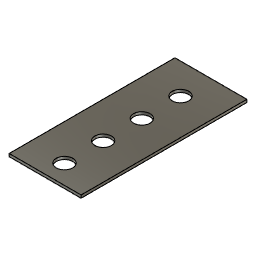
Untitled v1 (Autodesk Fusion 360 design; units mm, degrees)
Autodesk Fusion 360 part; units mm, degrees
sketch "Sketch1" plane through (0, 0, 0) normal (0, 0, 1) x (1, 0, 0)
  line L0 (6.508, 15) -> (-6.508, 15)
  line L1 (-6.508, 15) -> (-6.508, -15)
  line L2 (-6.508, -15) -> (6.508, -15)
  line L3 (6.508, -15) -> (6.508, 15)
  line L4 (6.508, 15) -> (-6.508, -15) construction
  line L5 (-6.508, 15) -> (6.508, -15) construction
  line L6 (0, 15) -> (0, -15) construction
  circle A0 centre (0, 13) radius 2
  circle A1 centre (0, 9.5) radius 1.5
  circle A2 centre (0, 6) radius 2
  circle A3 centre (0, 2.5) radius 1.5
  circle A4 centre (0, -1) radius 2
  circle A5 centre (0, -4.5) radius 1.5
  circle A6 centre (0, -8) radius 2
  circle A7 centre (0, -11.5) radius 1.5
  dimension "d1" = 13.016
  dimension "d2" = 30
  dimension "d3" = 4
  dimension "d4" = 3
  dimension "d5" = 4
  dimension "d6" = 3
  dimension "d7" = 4
  dimension "d8" = 3
  dimension "d9" = 4
  dimension "d10" = 3
  constraint horizontal L0
  constraint perpendicular L0 L1
  constraint parallel L0 L2
  constraint parallel L1 L3
  constraint coincident L4 origin
  constraint coincident L5 origin
  constraint midpoint L0 L6.start
  constraint midpoint L2 L6.end
  constraint coincident L6.start A0
  measures "d1" distance of L1.end L2.end
  measures "d2" distance of L0.end L1.end
  measures "d3" diameter of A0
  measures "d4" diameter of A1
  measures "d5" diameter of A2
  measures "d6" diameter of A3
  measures "d7" diameter of A4
  measures "d8" diameter of A5
  measures "d9" diameter of A6
  measures "d10" diameter of A7
extrude "Extrude1" add sketch "Sketch1" along normal blind 0.5 contours A6 | A4 | A2 | A0 | L0 L1 L2 L3
